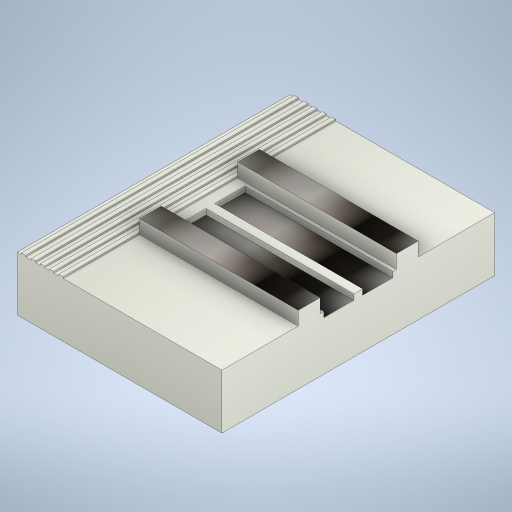
# Autodesk Inventor part: 門
Saved by Autodesk Inventor 2024.2 (Build 282272000, 272)
## iProperties
Created: 2024-06-05
Part Number: 門
Material: 一般
Document SubType Name: Modeling
Designer: sohil
Density: 1 g/cm^3
Appearance: 預設
Author: sohil
Autodesk Inventor part; units mm, degrees
ref_plane "YZ Plane" through (0, 0, 0) normal (1, 0, 0) x (0, 1, 0)
ref_plane "XZ Plane" through (0, 0, 0) normal (0, 1, 0) x (-1, 0, 0)
ref_plane "XY Plane" through (0, 0, 0) normal (0, 0, 1) x (1, 0, 0)
sketch "草圖1" plane through (0, 0, 0) normal (0, 1, 0) x (-1, 0, 0)
  line L0 (2.7779, 3.5245) -> (-4.7221, 3.5245)
  line L1 (-4.7221, 3.5245) -> (-4.7221, -6.4755)
  line L2 (-4.7221, -6.4755) -> (2.7779, -6.4755)
  line L3 (2.7779, -6.4755) -> (2.7779, 3.5245)
  line L4 (1.1026, 3.5245) -> (1.1026, -6.4755)
  line L5 (1.1026, 0.7245) -> (-4.7221, 0.7245)
  line L6 (1.1026, -0.0755) -> (-4.7221, -0.0755)
  line L7 (1.1026, -2.8755) -> (-4.7221, -2.8755)
  line L8 (1.1026, -3.6755) -> (-4.7221, -3.6755)
  line L9 (1.1026, -1.4755) -> (-4.7221, -1.4755)
  line L10 (0.6975, -1.6358) -> (-3.8571, -1.6358)
  line L11 (-3.8571, -1.6358) -> (-3.8571, -2.7441)
  line L12 (-3.8571, -2.7441) -> (0.6975, -2.7441)
  line L13 (0.6975, -2.7441) -> (0.6975, -1.6358)
  line L14 (0.6975, -1.3152) -> (-3.8571, -1.3152)
  line L15 (-3.8571, -1.3152) -> (-3.8571, -0.207)
  line L16 (-3.8571, -0.207) -> (0.6975, -0.207)
  line L17 (0.6975, -0.207) -> (0.6975, -1.3152)
  line L18 (1.4446, 3.5245) -> (1.4446, -6.4755)
  line L19 (1.2626, 3.5245) -> (1.2626, -6.4755)
  line L20 (1.6046, 3.5245) -> (1.6046, -6.4755)
  line L21 (1.9385, 3.5245) -> (1.9385, -6.4755)
  line L22 (1.7785, 3.5245) -> (1.7785, -6.4755)
  line L23 (2.106, 3.5245) -> (2.106, -6.4755)
  line L24 (2.266, 3.5245) -> (2.266, -6.4755)
  line L25 (2.6263, 3.5245) -> (2.6263, -6.4755)
  line L26 (2.4663, 3.5245) -> (2.4663, -6.4755)
  line L27 (-3.8571, -0.207) -> (-3.8571, -1.3152)
  line L28 (-3.8571, -1.3152) -> (-4.7221, -1.3152)
  line L29 (-4.7221, -1.3152) -> (-4.7221, -0.207)
  line L30 (-4.7221, -0.207) -> (-3.8571, -0.207)
  line L31 (-3.8571, -1.6358) -> (-3.8571, -2.7441)
  line L32 (-3.8571, -2.7441) -> (-4.7221, -2.7441)
  line L33 (-4.7221, -2.7441) -> (-4.7221, -1.6358)
  line L34 (-4.7221, -1.6358) -> (-3.8571, -1.6358)
  line L35 (-3.8571, -0.207) -> (-3.8571, -1.3152)
  line L36 (-3.8571, -1.3152) -> (-4.7221, -1.3152)
  line L37 (-4.7221, -1.3152) -> (-4.7221, -0.207)
  line L38 (-4.7221, -0.207) -> (-3.8571, -0.207)
  line L39 (-3.8571, -1.6358) -> (-3.8571, -2.7441)
  line L40 (-3.8571, -2.7441) -> (-4.7221, -2.7441)
  line L41 (-4.7221, -2.7441) -> (-4.7221, -1.6358)
  line L42 (-4.7221, -1.6358) -> (-3.8571, -1.6358)
  point P0 (0, 0)
  dimension "d0" = 7.5
  dimension "d1" = 10
  dimension "d2" = 0.8
  dimension "d3" = 0.8
  dimension "d4" = 2.8
  dimension "d5" = 2.8
  dimension "d14" = 0.16
  dimension "d15" = 1.6753
  dimension "d16" = 0.16
  dimension "d17" = 0.16
  dimension "d18" = 0.16
  dimension "d19" = 0.16
  constraints: 82 end point, 15 equal length, 10 perpendicular, 10 vertical, 8 point on line, 4 symmetric about line, 2 midpoint, 1 horizontal, 26 other
  measures "d0" distance of L3.start L1.end
  measures "d1" distance of L1.end L1.start
  measures "d2" distance between parallel lines of L6 L5
  measures "d3" distance between parallel lines of L8 L7
  measures "d5" distance between parallel lines of L7 L6
  measures "d14" distance between parallel lines of L4 L19
  measures "d15" distance between parallel lines of L4 L3
  measures "d16" distance between parallel lines of L26 L25
  measures "d17" distance between parallel lines of L24 L23
  measures "d18" distance between parallel lines of L21 L22
  measures "d19" distance between parallel lines of L20 L18
extrude "擠出1" add sketch "草圖1" along normal blind 2 contours L3 L2 L25 L0 | L26 L2 L24 L0 | L23 L2 L21 L0 | L22 L2 L20 L0 | L18 L2 L19 L0 | L4 L5 L1 L0 | L2 L1 L8 L4
extrude "擠出2" add sketch "草圖1" along normal blind 2.5 contours L4 L6 L1 L5 | L8 L1 L7 L4
extrude "擠出3" add sketch "草圖1" along normal blind 2 contours L4 L9 L1 L28 L14 L17 L16 L30 L6 | L4 L7 L1 L32 L12 L13 L10 L34 L9
extrude "擠出4" add sketch "草圖1" along normal blind 1.8 contours L30 L15 L28 L1 | L16 L17 L14 L15 | L34 L11 L32 L1 | L10 L13 L12 L11
extrude "擠出5" add sketch "草圖1" along normal blind 2.05 contours L25 L2 L26 L0 | L24 L2 L23 L0 | L21 L2 L22 L0 | L20 L2 L18 L0 | L19 L2 L4 L0
